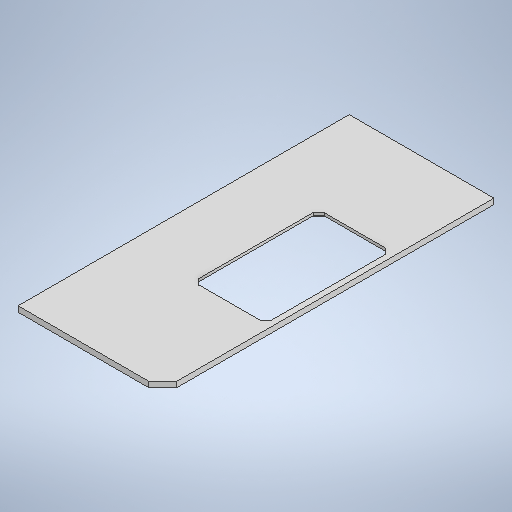
# Autodesk Inventor part: Part6
Saved by Autodesk Inventor 2025.2 (Build 292293000, 293)
## iProperties
Created: 2025-06-06
Part Number: Part6
Material: Generic
Document SubType Name: Sheet Metal
Designer: ziyuz
Density: 1 g/cm^3
Sheet Metal Rule: Default_mm
Appearance: Default
Author: ziyuz
Autodesk Inventor part; units mm, degrees
(part 1 of 2)
ref_plane "YZ Plane" through (0, 0, 0) normal (1, 0, 0) x (0, 1, 0)
ref_plane "XZ Plane" through (0, 0, 0) normal (0, 1, 0) x (-1, 0, 0)
ref_plane "XY Plane" through (0, 0, 0) normal (0, 0, 1) x (1, 0, 0)
sketch "Sketch1" plane through (0, 0, 0) normal (0, 1, 0) x (-1, 0, 0)
  line L0 (-29.0932, -58.6501) -> (-29.0932, -48.6501)
  line L1 (-29.0932, -58.6501) -> (-29.0932, 55.3499)
  line L2 (-29.0932, 55.3499) -> (-24.0932, 60.3499)
  line L3 (-29.0932, 55.3499) -> (-24.0932, 60.3499)
  line L4 (-24.0932, 60.3499) -> (22.9068, 60.3499)
  line L5 (-24.0932, 60.3499) -> (22.9068, 60.3499)
  line L6 (22.9068, 60.3499) -> (22.9068, -58.6501)
  line L7 (22.9068, -58.6501) -> (-29.0932, -58.6501)
  line L8 (-29.0932, -38.6501) -> (0.9068, -38.6501)
  line L9 (-29.0932, -38.6501) -> (2.9068, -38.6501)
  line L10 (2.9068, -38.6501) -> (2.9068, 31.3499)
  line L11 (2.9068, 31.3499) -> (-29.0932, 31.3499)
  line L12 (-29.0932, -38.6501) -> (-29.0932, -23.6501)
  line L13 (-29.0932, -23.6501) -> (2.9068, -23.6501)
  line L14 (-29.0932, 31.3499) -> (-29.0932, 21.3499)
  line L15 (-29.0932, 21.3499) -> (2.9068, 21.3499)
  line L16 (-29.0932, -23.6501) -> (-29.0932, 21.3499)
  line L17 (-29.0932, -23.6501) -> (-27.0932, -23.6501)
  line L18 (-27.0932, -23.6501) -> (-27.0932, 21.3499)
  line L19 (-29.0932, 21.3499) -> (-27.0932, 21.3499)
  line L20 (0.9068, -38.6501) -> (0.9068, 31.3499)
  line L21 (0.9068, -23.6501) -> (-1.0932, -23.6501)
  line L22 (-1.0932, -23.6501) -> (-1.0932, 21.3499)
  point P0 (0, 0)
  point P1 (-27.0932, 58.3499)
  dimension "d0" = 32
  dimension "d1" = 70
  dimension "d2" = 15
  dimension "d3" = 10
  dimension "d4" = 2
  dimension "d5" = 2
  constraints: 46 end point, 11 point on line, 8 perpendicular, 5 collinear, 1 vertical
  measures "d0" distance of L8.start L9.end
  measures "d1" distance of L9.end L10.end
  measures "d2" distance of L8.start L12.end
  measures "d3" distance of L11.end L14.end
  measures "d4" distance of L12.end L17.end
  measures "d5" distance of L21.start L21.end
extrude "Extrusion1" add sketch "Sketch1" along normal blind 2 contours L0 L1 L8 L9 L10 L11 L2 L4 L6 L7 | L1 L13 L20 L8 | L1 L15 L18 L13 | L20 L13 L10 L9 | L1 L11 L20 L15 | L20 L15 L10 L13 | L13 L22 L15 L20 | L20 L11 L10 L15
chamfer "Chamfer1" distance 2 angle 45 4 edges at (27.0932, 1, 21.3499) (27.0932, 1, -23.6501) (1.0932, 1, -23.6501) (1.0932, 1, 21.3499)
chamfer "Chamfer2" distance 1 angle 45 8 edges at (14.0932, 0, -23.6501) (2.0932, 0, -22.6501) (1.0932, 0, -1.1501) (2.0932, 0, 20.3499) (14.0932, 0, 21.3499) (26.0932, 0, 20.3499) (27.0932, 0, -1.1501) (26.0932, 0, -22.6501)
sketch "Sketch2" plane through (0, 0, 0) normal (0, -1, 0) x (1, 0, 0)
  line L0 (22.5848, 53.3001) -> (22.5848, 27.0796) construction
  line L1 (22.5848, 27.0796) -> (14.0309, 27.0796) construction
  line L2 (14.0309, 27.0796) -> (14.0309, 53.3001) construction
  line L3 (14.0309, 53.3001) -> (22.5848, 53.3001) construction
  line L4 (23.1405, -28.7557) -> (23.1405, -54.9763) construction
  line L5 (23.1405, -54.9763) -> (14.5866, -54.9763) construction
  line L6 (14.5866, -54.9763) -> (14.5866, -28.7557) construction
  line L7 (14.5866, -28.7557) -> (23.1405, -28.7557) construction
  line L8 (-13.0132, 54.473) -> (-4.4593, 54.473) construction
  line L9 (-4.4593, 54.473) -> (-4.4593, -53.9023) construction
  line L10 (-4.4593, -53.9023) -> (-13.0132, -53.9023) construction
  line L11 (-13.0132, -53.9023) -> (-13.0132, 54.473) construction
  line L12 (-24.1819, 54.7415) -> (-15.628, 54.7415) construction
  line L13 (-15.628, 54.7415) -> (-15.628, -53.6339) construction
  line L14 (-15.628, -53.6339) -> (-24.1819, -53.6339) construction
  line L15 (-24.1819, -53.6339) -> (-24.1819, 54.7415) construction
  line L16 (16.4848, 43.7144) -> (16.4848, 45.6962)
  line L17 (16.4848, 45.6962) -> (16.8688, 45.6962)
  line L18 (16.8688, 45.6962) -> (16.8688, 45.299)
  spline S0 degree 2 poles (16.8688, 45.299) (16.8688, 45.1621) (16.9571, 45.0739) (17.0586, 45.0739) knots 0 0 0 1 2 2 2
  line L19 (17.0586, 45.0739) -> (21.9095, 45.0739)
  spline S1 degree 2 poles (21.9095, 45.0739) (22.1478, 45.0739) (22.1655, 45.0915) (22.1655, 45.299) knots 0 0 0 1 2 2 2
  spline S2 degree 2 poles (22.1655, 45.299) (22.1655, 45.7448) (21.8565, 46.0846) (21.0576, 46.3804) knots 0 0 0 1 2 2 2
  line L20 (21.0576, 46.3804) -> (21.1105, 46.7379)
  line L21 (21.1105, 46.7379) -> (22.5848, 46.4069)
  line L22 (22.5848, 46.4069) -> (22.5848, 42.9684)
  line L23 (22.5848, 42.9684) -> (21.115, 42.6727)
  line L24 (21.115, 42.6727) -> (21.0576, 42.9949)
  spline S3 degree 2 poles (21.0576, 42.9949) (21.8256, 43.2951) (22.1655, 43.5687) (22.1655, 44.0145) knots 0 0 0 1 2 2 2
  spline S4 degree 2 poles (22.1655, 44.0145) (22.1655, 44.3191) (22.1478, 44.3367) (21.8742, 44.3367) knots 0 0 0 1 2 2 2
  line L25 (21.8742, 44.3367) -> (17.0586, 44.3367)
  spline S5 degree 2 poles (17.0586, 44.3367) (16.9571, 44.3367) (16.8688, 44.2264) (16.8688, 44.1161) knots 0 0 0 1 2 2 2
  line L26 (16.8688, 44.1161) -> (16.8688, 43.7144)
  line L27 (16.8688, 43.7144) -> (16.4848, 43.7144)
  spline S6 degree 2 poles (22.011, 41.7237) (22.1125, 41.7237) (22.2008, 41.812) (22.2008, 41.9488) knots 0 0 0 1 2 2 2
  line L28 (22.2008, 41.9488) -> (22.2008, 42.2446)
  line L29 (22.2008, 42.2446) -> (22.5848, 42.2446)
  line L30 (22.5848, 42.2446) -> (22.5848, 40.5982)
  spline S7 degree 2 poles (22.5848, 40.5982) (22.5848, 39.4859) (21.1414, 38.1529) (19.654, 38.1529) knots 0 0 0 1 2 2 2
  spline S8 degree 2 poles (19.654, 38.1529) (18.0297, 38.1529) (16.4848, 39.4462) (16.4848, 40.7041) knots 0 0 0 1 2 2 2
  line L31 (16.4848, 40.7041) -> (16.4848, 42.2799)
  line L32 (16.4848, 42.2799) -> (16.8688, 42.2799)
  line L33 (16.8688, 42.2799) -> (16.8688, 41.9488)
  spline S9 degree 2 poles (16.8688, 41.9488) (16.8688, 41.812) (16.9571, 41.7237) (17.0586, 41.7237) knots 0 0 0 1 2 2 2
  line L34 (17.0586, 41.7237) -> (22.011, 41.7237)
  spline S10 degree 2 poles (19.5878, 38.9915) (21.0443, 38.9915) (22.2008, 39.8478) (22.2008, 40.5938) knots 0 0 0 1 2 2 2
  spline S11 degree 2 poles (22.2008, 40.5938) (22.2008, 40.81) (22.0993, 40.9866) (22.011, 40.9866) knots 0 0 0 1 2 2 2
  line L35 (22.011, 40.9866) -> (17.0586, 40.9866)
  spline S12 degree 2 poles (17.0586, 40.9866) (16.9659, 40.9866) (16.8688, 40.8454) (16.8688, 40.6997) knots 0 0 0 1 2 2 2
  spline S13 degree 2 poles (16.8688, 40.6997) (16.8688, 39.9802) (17.959, 38.9915) (19.5878, 38.9915) knots 0 0 0 1 2 2 2
  spline S14 degree 2 poles (22.011, 35.403) (22.1125, 35.403) (22.2008, 35.4913) (22.2008, 35.6281) knots 0 0 0 1 2 2 2
  line L36 (22.2008, 35.6281) -> (22.2008, 36.5462)
  line L37 (22.2008, 36.5462) -> (22.5848, 36.5462)
  line L38 (22.5848, 36.5462) -> (22.5848, 33.5227)
  line L39 (22.5848, 33.5227) -> (22.2008, 33.5227)
  line L40 (22.2008, 33.5227) -> (22.2008, 34.4452)
  spline S15 degree 2 poles (22.2008, 34.4452) (22.2008, 34.5511) (22.1125, 34.6659) (22.011, 34.6659) knots 0 0 0 1 2 2 2
  line L41 (22.011, 34.6659) -> (17.0939, 34.6659)
  spline S16 degree 2 poles (17.0939, 34.6659) (16.295, 34.6659) (15.3769, 35.6899) (15.3769, 36.4535) knots 0 0 0 1 2 2 2
  spline S17 degree 2 poles (15.3769, 36.4535) (15.3769, 37.0053) (15.8359, 37.6144) (16.1582, 37.6144) knots 0 0 0 1 2 2 2
  spline S18 degree 2 poles (16.1582, 37.6144) (16.4053, 37.6144) (16.6613, 37.3142) (16.6613, 37.1421) knots 0 0 0 1 2 2 2
  spline S19 degree 2 poles (16.6613, 37.1421) (16.6613, 36.9302) (16.3612, 36.6698) (16.1582, 36.6698) knots 0 0 0 1 2 2 2
  spline S20 degree 2 poles (16.1582, 36.6698) (16.0787, 36.6698) (15.9375, 36.7184) (15.9022, 36.7757) knots 0 0 0 1 2 2 2
  spline S21 degree 2 poles (15.9022, 36.7757) (15.8801, 36.736) (15.7962, 36.5065) (15.7962, 36.3123) knots 0 0 0 1 2 2 2
  spline S22 degree 2 poles (15.7962, 36.3123) (15.7962, 35.9018) (16.3303, 35.403) (17.0939, 35.403) knots 0 0 0 1 2 2 2
  line L42 (17.0939, 35.403) -> (22.011, 35.403)
  line L43 (6.459, 44.9194) -> (6.075, 44.9194)
  line L44 (6.075, 44.9194) -> (6.075, 46.7644)
  line L45 (6.075, 46.7644) -> (6.459, 46.7644)
  line L46 (6.459, 46.7644) -> (6.459, 46.4378)
  spline S23 degree 2 poles (6.459, 46.4378) (6.459, 46.3009) (6.5473, 46.2126) (6.6488, 46.2126) knots 0 0 0 1 2 2 2
  line L47 (6.6488, 46.2126) -> (11.6012, 46.2126)
  spline S24 degree 2 poles (11.6012, 46.2126) (11.7027, 46.2126) (11.791, 46.3009) (11.791, 46.4378) knots 0 0 0 1 2 2 2
  line L48 (11.791, 46.4378) -> (11.791, 46.7335)
  line L49 (11.791, 46.7335) -> (12.175, 46.7335)
  line L50 (12.175, 46.7335) -> (12.175, 42.9773)
  line L51 (12.175, 42.9773) -> (10.789, 42.5359)
  line L52 (10.789, 42.5359) -> (10.6831, 42.8448)
  spline S25 degree 2 poles (10.6831, 42.8448) (11.2657, 43.1494) (11.791, 43.8689) (11.791, 44.2882) knots 0 0 0 1 2 2 2
  line L53 (11.791, 44.2882) -> (11.791, 45.2548)
  spline S26 degree 2 poles (11.791, 45.2548) (11.791, 45.3608) (11.6983, 45.4755) (11.6012, 45.4755) knots 0 0 0 1 2 2 2
  line L54 (11.6012, 45.4755) -> (9.4737, 45.4755)
  line L55 (9.4737, 45.4755) -> (9.4737, 44.4294)
  spline S27 degree 2 poles (9.4737, 44.4294) (9.4737, 44.1205) (9.7341, 43.86) (10.0431, 43.86) knots 0 0 0 1 2 2 2
  line L56 (10.0431, 43.86) -> (10.3035, 43.86)
  line L57 (10.3035, 43.86) -> (10.3035, 43.4716)
  line L58 (10.3035, 43.4716) -> (8.1186, 43.4716)
  line L59 (8.1186, 43.4716) -> (8.1186, 43.86)
  line L60 (8.1186, 43.86) -> (8.3437, 43.86)
  spline S28 degree 2 poles (8.3437, 43.86) (8.7322, 43.86) (9.0897, 44.1293) (9.0897, 44.4294) knots 0 0 0 1 2 2 2
  line L61 (9.0897, 44.4294) -> (9.0897, 45.4755)
  line L62 (9.0897, 45.4755) -> (6.6488, 45.4755)
  spline S29 degree 2 poles (6.6488, 45.4755) (6.5473, 45.4755) (6.459, 45.3608) (6.459, 45.2548) knots 0 0 0 1 2 2 2
  line L63 (6.459, 45.2548) -> (6.459, 44.9194)
  line L64 (8.8469, 40.9513) -> (6.6488, 40.9513)
  spline S30 degree 2 poles (6.6488, 40.9513) (6.5473, 40.9513) (6.459, 40.8365) (6.459, 40.7306) knots 0 0 0 1 2 2 2
  line L65 (6.459, 40.7306) -> (6.459, 40.3951)
  line L66 (6.459, 40.3951) -> (6.075, 40.3951)
  line L67 (6.075, 40.3951) -> (6.075, 42.2401)
  line L68 (6.075, 42.2401) -> (6.459, 42.2401)
  line L69 (6.459, 42.2401) -> (6.459, 41.9135)
  spline S31 degree 2 poles (6.459, 41.9135) (6.459, 41.7767) (6.5473, 41.6884) (6.6488, 41.6884) knots 0 0 0 1 2 2 2
  line L70 (6.6488, 41.6884) -> (11.6012, 41.6884)
  spline S32 degree 2 poles (11.6012, 41.6884) (11.7027, 41.6884) (11.791, 41.7767) (11.791, 41.9135) knots 0 0 0 1 2 2 2
  line L71 (11.791, 41.9135) -> (11.791, 42.2092)
  line L72 (11.791, 42.2092) -> (12.175, 42.2092)
  line L73 (12.175, 42.2092) -> (12.175, 40.0773)
  spline S33 degree 2 poles (12.175, 40.0773) (12.175, 39.1769) (11.2569, 38.1838) (10.5639, 38.1838) knots 0 0 0 1 2 2 2
  spline S34 degree 2 poles (10.5639, 38.1838) (9.7253, 38.1838) (8.8469, 39.2431) (8.8469, 39.9714) knots 0 0 0 1 2 2 2
  line L74 (8.8469, 39.9714) -> (8.8469, 40.9513)
  spline S35 degree 2 poles (9.2309, 40.1789) (9.2309, 39.6889) (9.8092, 38.9518) (10.5286, 38.9518) knots 0 0 0 1 2 2 2
  spline S36 degree 2 poles (10.5286, 38.9518) (11.1819, 38.9518) (11.791, 39.5609) (11.791, 40.2495) knots 0 0 0 1 2 2 2
  line L75 (11.791, 40.2495) -> (11.791, 40.7306)
  spline S37 degree 2 poles (11.791, 40.7306) (11.791, 40.8365) (11.6983, 40.9513) (11.6012, 40.9513) knots 0 0 0 1 2 2 2
  line L76 (11.6012, 40.9513) -> (9.2309, 40.9513)
  line L77 (9.2309, 40.9513) -> (9.2309, 40.1789)
  line L78 (6.075, 34.6659) -> (6.075, 36.6477)
  line L79 (6.075, 36.6477) -> (6.459, 36.6477)
  line L80 (6.459, 36.6477) -> (6.459, 36.2505)
  spline S38 degree 2 poles (6.459, 36.2505) (6.459, 36.1137) (6.5473, 36.0254) (6.6488, 36.0254) knots 0 0 0 1 2 2 2
  line L81 (6.6488, 36.0254) -> (11.4997, 36.0254)
  spline S39 degree 2 poles (11.4997, 36.0254) (11.738, 36.0254) (11.7557, 36.043) (11.7557, 36.2505) knots 0 0 0 1 2 2 2
  spline S40 degree 2 poles (11.7557, 36.2505) (11.7557, 36.6963) (11.4467, 37.0362) (10.6478, 37.3319) knots 0 0 0 1 2 2 2
  line L82 (10.6478, 37.3319) -> (10.7008, 37.6894)
  line L83 (10.7008, 37.6894) -> (12.175, 37.3584)
  line L84 (12.175, 37.3584) -> (12.175, 33.92)
  line L85 (12.175, 33.92) -> (10.7052, 33.6242)
  line L86 (10.7052, 33.6242) -> (10.6478, 33.9464)
  spline S41 degree 2 poles (10.6478, 33.9464) (11.4158, 34.2466) (11.7557, 34.5202) (11.7557, 34.9661) knots 0 0 0 1 2 2 2
  spline S42 degree 2 poles (11.7557, 34.9661) (11.7557, 35.2706) (11.738, 35.2883) (11.4644, 35.2883) knots 0 0 0 1 2 2 2
  line L87 (11.4644, 35.2883) -> (6.6488, 35.2883)
  spline S43 degree 2 poles (6.6488, 35.2883) (6.5473, 35.2883) (6.459, 35.1779) (6.459, 35.0676) knots 0 0 0 1 2 2 2
  line L88 (6.459, 35.0676) -> (6.459, 34.6659)
  line L89 (6.459, 34.6659) -> (6.075, 34.6659)
  point P0 (0, 0)
  constraints: 8 other
extrude "Extrusion2" add sketch "Sketch2" along normal blind 0.5
sketch "Sketch4" plane through (0, 0, 0) normal (0, -1, 0) x (1, 0, 0)
  line L0 (23.6842, -29.6175) -> (23.6842, -52.515) construction
  line L1 (23.6842, -52.515) -> (1.0923, -52.515) construction
  line L2 (1.0923, -52.515) -> (1.0923, -29.6175) construction
  line L3 (1.0923, -29.6175) -> (23.6842, -29.6175) construction
  spline S0 degree 2 poles (18.1434, -33.7347) (18.3329, -33.7347) (18.5408, -33.9796) (18.5408, -34.3262) (18.4761, -34.6543) (18.3699, -34.7976) knots 0 0 0 1 2 3 4 4 4
  line L4 (18.3699, -34.7976) -> (18.3699, -35.1765)
  spline S1 degree 2 poles (18.3699, -35.1765) (18.3606, -35.2967) (18.3606, -35.403) knots 0 0 0 1 1 1
  line L5 (18.3606, -35.403) -> (18.3606, -35.5555)
  spline S2 degree 2 poles (18.3606, -35.5555) (18.3606, -35.7496) (18.3375, -36.2764) (18.393, -36.8078) (18.5639, -37.2792) (18.7627, -37.4224) knots 0 0 0 1 2 3 4 4 4
  spline S3 degree 2 poles (18.7627, -37.4224) (18.7072, -37.3716) (18.7026, -37.2653) (18.7026, -37.196) knots 0 0 0 1 2 2 2
  line L6 (18.7026, -37.196) -> (18.7026, -37.0851)
  line L7 (18.7026, -37.0851) -> (18.7534, -36.9187)
  spline S4 degree 2 poles (18.7534, -36.9187) (18.7904, -36.7986) (18.8828, -36.5352) (18.929, -36.415) knots 0 0 0 1 2 2 2
  line L8 (18.929, -36.415) -> (18.9799, -36.2487)
  spline S5 degree 2 poles (18.9799, -36.2487) (18.9937, -36.2117) (19.1, -35.976) (19.1693, -35.842) knots 0 0 0 1 2 2 2
  line L9 (19.1693, -35.842) -> (19.2895, -35.5832)
  spline S6 degree 2 poles (19.2895, -35.5832) (19.3403, -35.463) (19.3727, -35.4122) knots 0 0 0 1 1 1
  spline S7 degree 2 poles (19.3727, -35.4122) (19.3865, -35.3799) (19.4928, -35.1996) (19.6222, -34.9824) (19.7331, -34.793) (19.7655, -34.7468) knots 0 0 0 1 2 3 4 4 4
  spline S8 degree 2 poles (19.7655, -34.7468) (19.8302, -34.6312) (20.052, -34.3262) (20.3154, -34.0443) (20.6065, -33.8502) (20.7683, -33.8502) knots 0 0 0 1 2 3 4 4 4
  spline S9 degree 2 poles (20.7683, -33.8502) (20.9947, -33.8502) (21.2442, -34.1414) (21.272, -34.354) knots 0 0 0 1 2 2 2
  spline S10 degree 2 poles (21.272, -34.354) (21.2812, -34.4094) (21.2951, -34.5573) knots 0 0 0 1 1 1
  line L10 (21.2951, -34.5573) -> (21.3321, -34.9224)
  spline S11 degree 2 poles (21.3321, -34.9224) (21.3459, -35.1303) (21.3783, -35.3706) knots 0 0 0 1 1 1
  line L11 (21.3783, -35.3706) -> (21.4245, -35.842)
  spline S12 degree 2 poles (21.4245, -35.842) (21.4383, -36.073) (21.4753, -36.4659) (21.5077, -36.7062) (21.711, -36.8818) (21.8311, -36.9187) knots 0 0 0 1 2 3 4 4 4
  line L12 (21.8311, -36.9187) -> (22.8339, -37.7043)
  spline S13 degree 2 poles (22.8339, -37.7043) (22.8709, -37.7413) (22.9033, -37.8984) (22.9033, -37.9446) knots 0 0 0 1 2 2 2
  spline S14 degree 2 poles (22.9033, -37.9446) (22.6907, -37.9446) (22.3349, -37.7644) (22.0206, -37.5426) (21.7572, -37.3624) (21.6324, -37.3624) knots 0 0 0 1 2 3 4 4 4
  spline S15 degree 2 poles (21.6324, -37.3624) (21.5816, -37.3624) (21.5492, -37.4224) knots 0 0 0 1 1 1
  spline S16 degree 2 poles (21.5492, -37.4224) (21.5677, -37.2884) (21.3783, -37.1359) (21.138, -37.0158) (20.9254, -36.8679) (20.9254, -36.7293) knots 0 0 0 1 2 3 4 4 4
  spline S17 degree 2 poles (20.9254, -36.7293) (20.9254, -36.6415) (20.9947, -36.5814) (21.1056, -36.5814) (21.2489, -36.6091) (21.3228, -36.6091) knots 0 0 0 1 2 3 4 4 4
  line L13 (21.3228, -36.6091) -> (21.3228, -36.5259)
  line L14 (21.3228, -36.5259) -> (20.8191, -34.7468)
  spline S18 degree 2 poles (20.8191, -34.7468) (20.7498, -34.6867) (20.6389, -34.5434) (20.6019, -34.4695) knots 0 0 0 1 2 2 2
  spline S19 degree 2 poles (20.6019, -34.4695) (20.5095, -34.5896) (20.3154, -34.8762) (20.1352, -35.1858) (19.9734, -35.4862) (19.9318, -35.6387) knots 0 0 0 1 2 3 4 4 4
  spline S20 degree 2 poles (19.9318, -35.6387) (19.8717, -35.8189) (19.7424, -36.2255) (19.5806, -36.623) (19.3865, -36.9927) (19.2571, -37.1452) knots 0 0 0 1 2 3 4 4 4
  spline S21 degree 2 poles (19.2571, -37.1452) (19.2063, -37.2052) (19.0538, -37.4086) (18.8874, -37.6119) (18.7072, -37.7644) (18.624, -37.7644) knots 0 0 0 1 2 3 4 4 4
  spline S22 degree 2 poles (18.624, -37.7644) (18.4068, -37.7644) (18.1942, -37.538) (18.0649, -37.2376) (17.9447, -36.9418) (17.8107, -36.8679) knots 0 0 0 1 2 3 4 4 4
  spline S23 degree 2 poles (17.8107, -36.8679) (17.6074, -36.3734) (17.4179, -35.3568) (17.4179, -34.8299) knots 0 0 0 1 2 2 2
  spline S24 degree 2 poles (17.4179, -34.8299) (17.4179, -34.6266) (17.4641, -34.2338) (17.6212, -33.9242) (17.9031, -33.7347) (18.1434, -33.7347) knots 0 0 0 1 2 3 4 4 4
  spline S25 degree 2 poles (21.8358, -38.9705) (21.882, -38.9798) (22.0483, -39.0168) knots 0 0 0 1 1 1
  line L15 (22.0483, -39.0168) -> (22.4088, -39.1138)
  spline S26 degree 2 poles (22.4088, -39.1138) (22.6075, -39.1739) (22.9772, -39.2802) (23.065, -39.3079) knots 0 0 0 1 2 2 2
  line L16 (23.065, -39.3079) -> (23.1482, -39.3495)
  spline S27 degree 2 poles (23.1482, -39.3495) (23.2267, -39.3865) (23.3099, -39.4234) knots 0 0 0 1 1 1
  line L17 (23.3099, -39.4234) -> (23.4902, -39.5159)
  spline S28 degree 2 poles (23.4902, -39.5159) (23.578, -39.5574) (23.6704, -39.6129) (23.6842, -39.6591) (23.6842, -39.7007) knots 0 0 0 1 2 3 3 3
  spline S29 degree 2 poles (23.6842, -39.7007) (23.6842, -39.7099) (23.6796, -39.7238) knots 0 0 0 1 1 1
  line L18 (23.6796, -39.7238) -> (23.6796, -39.7562)
  spline S30 degree 2 poles (23.6796, -39.7562) (23.5641, -39.8209) (23.2406, -39.8902) (22.9171, -39.9225) (22.76, -39.9225) knots 0 0 0 1 2 3 3 3
  line L19 (22.76, -39.9225) -> (22.5105, -39.9225)
  spline S31 degree 2 poles (22.5105, -39.9225) (22.4319, -39.9502) (22.2886, -40.0473) (22.2286, -40.0889) knots 0 0 0 1 2 2 2
  line L20 (22.2286, -40.0889) -> (18.9429, -41.7063)
  spline S32 degree 2 poles (18.9429, -41.7063) (18.9336, -41.808) (18.9336, -41.979) (18.8967, -42.0945) (18.8042, -42.1592) (18.7164, -42.1592) knots 0 0 0 1 2 3 4 4 4
  spline S33 degree 2 poles (18.7164, -42.1592) (18.6471, -42.1592) (18.5778, -42.0991) (18.5593, -42.0621) knots 0 0 0 1 2 2 2
  line L21 (18.5593, -42.0621) -> (18.5131, -42.0021)
  spline S34 degree 2 poles (18.5131, -42.0021) (18.49, -41.979) (18.4346, -41.979) knots 0 0 0 1 1 1
  spline S35 degree 2 poles (18.4346, -41.979) (18.2867, -41.979) (18.0048, -42.0945) (17.7136, -42.2377) (17.4086, -42.3487) (17.2469, -42.3487) knots 0 0 0 1 2 3 4 4 4
  spline S36 degree 2 poles (17.2469, -42.3487) (17.2469, -42.2886) (17.2515, -42.1361) (17.3208, -42.0991) knots 0 0 0 1 2 2 2
  line L22 (17.3208, -42.0991) -> (18.5501, -41.4799)
  spline S37 degree 2 poles (18.5501, -41.4799) (18.5593, -41.1333) (18.5732, -40.8098) knots 0 0 0 1 1 1
  line L23 (18.5732, -40.8098) -> (18.5871, -40.2368)
  spline S38 degree 2 poles (18.5871, -40.2368) (18.5963, -39.9502) (18.6009, -39.7562) knots 0 0 0 1 1 1
  line L24 (18.6009, -39.7562) -> (18.6009, -39.5297)
  spline S39 degree 2 poles (18.6009, -39.5297) (18.5131, -39.4974) (18.1942, -39.4696) (17.8246, -39.4234) (17.4317, -39.3541) (17.1221, -39.2432) (16.9188, -39.063) (16.9188, -38.9243) knots 0 0 0 1 2 3 4 5 6 6 6
  spline S40 degree 2 poles (16.9188, -38.9243) (16.9188, -38.8735) (16.965, -38.7349) (17.0436, -38.6101) (17.1452, -38.5269) (17.2053, -38.5269) knots 0 0 0 1 2 3 4 4 4
  line L25 (17.2053, -38.5269) -> (18.49, -38.5269)
  line L26 (18.49, -38.5269) -> (21.8358, -38.9705)
  line L27 (18.9198, -39.5898) -> (18.9198, -39.9826)
  spline S41 degree 2 poles (18.9198, -39.9826) (18.9198, -40.1905) (18.9336, -40.6388) (18.966, -41.0732) (18.9937, -41.2627) knots 0 0 0 1 2 3 3 3
  line L28 (18.9937, -41.2627) -> (19.3264, -41.1518)
  line L29 (19.3264, -41.1518) -> (22.0576, -39.8763)
  line L30 (22.0576, -39.8763) -> (19.2155, -39.5898)
  line L31 (19.2155, -39.5898) -> (18.9198, -39.5898)
  spline S42 degree 2 poles (17.2977, -44.0909) (17.3717, -44.0585) (17.538, -44.0077) knots 0 0 0 1 1 1
  line L32 (17.538, -44.0077) -> (17.917, -43.8829)
  line L33 (17.917, -43.8829) -> (18.3514, -43.7581)
  spline S43 degree 2 poles (18.3514, -43.7581) (18.5778, -43.6888) (19.003, -43.5779) (19.3357, -43.4855) (19.4189, -43.4716) knots 0 0 0 1 2 3 3 3
  line L34 (19.4189, -43.4716) -> (19.8255, -43.3884)
  line L35 (19.8255, -43.3884) -> (20.3662, -43.2914)
  spline S44 degree 2 poles (20.3662, -43.2914) (20.662, -43.2452) (21.2627, -43.1481) (21.7849, -43.0696) (22.1546, -43.0234) (22.2055, -43.0234) knots 0 0 0 1 2 3 4 4 4
  line L36 (22.2055, -43.0234) -> (22.5983, -43.0234)
  spline S45 degree 2 poles (22.5983, -43.0234) (22.6445, -43.0234) (22.7138, -43.1666) (22.7508, -43.3561) (22.7646, -43.5455) (22.7646, -43.5825) knots 0 0 0 1 2 3 4 4 4
  line L37 (22.7646, -43.5825) -> (22.7646, -43.638)
  spline S46 degree 2 poles (22.7646, -43.638) (22.6445, -43.6796) (22.2655, -43.7627) (21.8912, -43.8459) (21.5585, -43.9522) (21.4846, -44.0308) knots 0 0 0 1 2 3 4 4 4
  line L38 (21.4846, -44.0308) -> (19.1, -46.4708)
  line L39 (19.1, -46.4708) -> (20.9254, -47.0438)
  spline S47 degree 2 poles (20.9254, -47.0438) (21.0086, -47.1039) (21.4152, -47.2333) (21.9189, -47.3858) (22.4735, -47.5337) (22.9217, -47.6862) (23.2175, -47.8387) (23.2175, -47.9034) knots 0 0 0 1 2 3 4 5 6 6 6
  spline S48 degree 2 poles (23.2175, -47.9034) (23.2175, -47.9449) (23.2083, -48.0327) (23.1574, -48.0466) knots 0 0 0 1 2 2 2
  line L40 (23.1574, -48.0466) -> (22.3718, -48.1621)
  spline S49 degree 2 poles (22.3718, -48.1621) (21.7387, -48.1529) (21.1426, -48.1621) knots 0 0 0 1 1 1
  line L41 (21.1426, -48.1621) -> (19.9503, -48.176)
  spline S50 degree 2 poles (19.9503, -48.176) (19.3634, -48.1899) (18.1942, -48.213) (17.5842, -48.213) knots 0 0 0 1 2 2 2
  spline S51 degree 2 poles (17.5842, -48.213) (17.5011, -48.213) (17.3486, -48.1852) (17.2977, -48.1021) knots 0 0 0 1 2 2 2
  spline S52 degree 2 poles (17.2977, -48.1021) (17.2885, -48.079) (17.2839, -47.9265) (17.2839, -47.9034) knots 0 0 0 1 2 2 2
  spline S53 degree 2 poles (17.2839, -47.9034) (17.2839, -47.8664) (17.2885, -47.7185) (17.2977, -47.7093) knots 0 0 0 1 2 2 2
  spline S54 degree 2 poles (17.2977, -47.7093) (17.307, -47.6862) (17.3671, -47.6122) (17.404, -47.5752) knots 0 0 0 1 2 2 2
  line L42 (17.404, -47.5752) -> (17.478, -47.5105)
  spline S55 degree 2 poles (17.478, -47.5105) (17.5103, -47.4921) (17.5242, -47.4921) knots 0 0 0 1 1 1
  line L43 (17.5242, -47.4921) -> (20.5326, -47.4921)
  line L44 (20.5326, -47.4921) -> (20.4817, -47.432)
  line L45 (20.4817, -47.432) -> (18.5778, -46.8728)
  spline S56 degree 2 poles (18.5778, -46.8728) (18.4946, -46.8497) (18.3514, -46.7296) (18.3514, -46.6325) knots 0 0 0 1 2 2 2
  spline S57 degree 2 poles (18.3514, -46.6325) (18.3514, -46.5863) (18.3699, -46.4662) (18.4161, -46.4246) knots 0 0 0 1 2 2 2
  spline S58 degree 2 poles (18.4161, -46.4246) (18.4207, -46.4199) (18.4761, -46.3876) knots 0 0 0 1 1 1
  line L46 (18.4761, -46.3876) -> (18.5778, -46.3368)
  line L47 (18.5778, -46.3368) -> (18.6841, -46.2905)
  line L48 (18.6841, -46.2905) -> (18.7442, -46.2628)
  spline S59 degree 2 poles (18.7442, -46.2628) (18.7534, -46.2628) (18.7904, -46.2166) (18.8042, -46.2074) knots 0 0 0 1 2 2 2
  spline S60 degree 2 poles (18.8042, -46.2074) (19.0399, -45.9209) (19.5621, -45.4079) (19.8302, -45.1584) knots 0 0 0 1 2 2 2
  line L49 (19.8302, -45.1584) -> (20.3616, -44.6639)
  spline S61 degree 2 poles (20.3616, -44.6639) (20.625, -44.4143) (20.8653, -44.1417) knots 0 0 0 1 1 1
  line L50 (20.8653, -44.1417) -> (20.759, -44.1417)
  line L51 (20.759, -44.1417) -> (19.9827, -44.2988)
  spline S62 degree 2 poles (19.9827, -44.2988) (19.576, -44.3912) (18.7211, -44.5391) (17.8708, -44.6454) (17.4641, -44.6454) knots 0 0 0 1 2 3 3 3
  line L52 (17.4641, -44.6454) -> (17.2469, -44.6454)
  spline S63 degree 2 poles (17.2469, -44.6454) (17.1406, -44.6177) (17.1175, -44.4652) (17.1175, -44.3912) knots 0 0 0 1 2 2 2
  spline S64 degree 2 poles (17.1175, -44.3912) (17.1175, -44.2849) (17.1683, -44.1324) (17.2977, -44.0909) knots 0 0 0 1 2 2 2
  line L53 (20.6851, -48.5365) -> (20.5696, -48.5365)
  line L54 (20.5696, -48.5365) -> (20.5696, -48.4348)
  line L55 (20.5696, -48.4348) -> (20.6851, -48.4348)
  line L56 (20.6851, -48.4348) -> (20.6851, -48.5365)
  line L57 (22.5983, -46.4246) -> (22.5382, -46.4246)
  line L58 (22.5382, -46.4246) -> (22.5382, -46.2628)
  line L59 (22.5382, -46.2628) -> (22.5983, -46.2628)
  line L60 (22.5983, -46.2628) -> (22.5983, -46.4246)
  spline S65 degree 2 poles (6.4292, -34.3748) (6.42, -34.2777) (6.4385, -33.871) (6.4893, -33.4551) (6.5817, -33.1409) (6.6464, -33.1409) knots 0 0 0 1 2 3 4 4 4
  spline S66 degree 2 poles (6.6464, -33.1409) (6.7666, -33.1409) (6.8729, -33.3904) (6.8729, -33.4875) knots 0 0 0 1 2 2 2
  spline S67 degree 2 poles (6.8729, -33.4875) (7.0993, -33.6123) (7.4551, -33.8618) (7.6215, -33.9912) knots 0 0 0 1 2 2 2
  line L61 (7.6215, -33.9912) -> (7.9542, -34.2638)
  spline S68 degree 2 poles (7.9542, -34.2638) (8.116, -34.3979) (8.3285, -34.5411) knots 0 0 0 1 1 1
  spline S69 degree 2 poles (8.3285, -34.5411) (8.8554, -34.9062) (9.8997, -35.6594) (10.4497, -35.9968) knots 0 0 0 1 2 2 2
  line L62 (10.4497, -35.9968) -> (10.4497, -35.8258)
  line L63 (10.4497, -35.8258) -> (10.0014, -33.3719)
  line L64 (10.0014, -33.3719) -> (10.0014, -33.1455)
  spline S70 degree 2 poles (10.0014, -33.1455) (10.0476, -33.1779) (10.1262, -33.3211) (10.177, -33.4782) (10.2001, -33.5476) knots 0 0 0 1 2 3 3 3
  line L65 (10.2001, -33.5476) -> (10.2232, -33.6538)
  line L66 (10.2232, -33.6538) -> (10.2232, -33.3119)
  line L67 (10.2232, -33.3119) -> (11.0088, -36.3295)
  spline S71 degree 2 poles (11.0088, -36.3295) (11.0597, -36.4035) (11.2353, -36.6669) (11.4063, -36.9719) (11.5264, -37.2815) (11.5264, -37.3924) knots 0 0 0 1 2 3 4 4 4
  line L68 (11.5264, -37.3924) -> (11.2861, -37.3924)
  line L69 (11.2861, -37.3924) -> (6.8497, -34.4117)
  line L70 (6.8497, -34.4117) -> (6.5956, -37.6697)
  line L71 (6.5956, -37.6697) -> (6.5956, -37.7159)
  line L72 (6.5956, -37.7159) -> (6.5817, -37.8083)
  spline S72 degree 2 poles (6.5817, -37.8083) (6.5632, -37.8545) (6.5216, -37.9377) (6.4893, -37.9516) knots 0 0 0 1 2 2 2
  line L73 (6.4893, -37.9516) -> (6.3738, -38.5107)
  line L74 (6.3738, -38.5107) -> (6.0364, -38.5107)
  spline S73 degree 2 poles (6.0364, -38.5107) (6.0364, -37.4848) (6.2536, -35.3637) (6.4292, -34.3748) knots 0 0 0 1 2 2 2
  spline S74 degree 2 poles (11.5588, -33.1455) (11.5588, -33.2888) (11.5033, -33.4274) (11.3554, -33.4274) knots 0 0 0 1 2 2 2
  spline S75 degree 2 poles (11.3554, -33.4274) (11.3554, -33.3211) (11.4294, -33.1455) (11.5588, -33.1455) knots 0 0 0 1 2 2 2
  spline S76 degree 2 poles (6.0595, -43.1181) (6.1335, -43.0118) (6.2536, -43.0072) knots 0 0 0 1 1 1
  line L75 (6.2536, -43.0072) -> (6.48, -43.0072)
  spline S77 degree 2 poles (6.48, -43.0072) (6.956, -43.0072) (7.8988, -43.0673) (8.3747, -43.0673) knots 0 0 0 1 2 2 2
  line L76 (8.3747, -43.0673) -> (8.7352, -43.0673)
  spline S78 degree 2 poles (8.7352, -43.0673) (8.6936, -42.8916) (8.6382, -42.5959) (8.6243, -42.3094) (8.6243, -42.1615) knots 0 0 0 1 2 3 3 3
  line L77 (8.6243, -42.1615) -> (8.6243, -41.8426)
  spline S79 degree 2 poles (8.6243, -41.8426) (8.6243, -41.4591) (8.7352, -40.7104) (8.7352, -40.3269) knots 0 0 0 1 2 2 2
  line L78 (8.7352, -40.3269) -> (8.6844, -40.3269)
  line L79 (8.6844, -40.3269) -> (6.6788, -40.8352)
  line L80 (6.6788, -40.8352) -> (6.1196, -40.8352)
  spline S80 degree 2 poles (6.1196, -40.8352) (6.0688, -40.8352) (5.9671, -40.6966) (5.8839, -40.5256) (5.8331, -40.35) (5.8331, -40.3223) knots 0 0 0 1 2 3 4 4 4
  spline S81 degree 2 poles (5.8331, -40.3223) (5.8331, -40.2298) (5.8793, -40.0866) (6.0087, -40.0496) knots 0 0 0 1 2 2 2
  line L81 (6.0087, -40.0496) -> (9.6872, -39.0976)
  spline S82 degree 2 poles (9.6872, -39.0976) (9.6964, -39.0976) (9.7981, -39.0838) knots 0 0 0 1 1 1
  line L82 (9.7981, -39.0838) -> (10.0338, -39.0468)
  line L83 (10.0338, -39.0468) -> (10.3064, -39.0144)
  spline S83 degree 2 poles (10.3064, -39.0144) (10.4404, -39.0006) (10.5236, -38.9913) knots 0 0 0 1 1 1
  spline S84 degree 2 poles (10.5236, -38.9913) (10.5329, -38.9913) (10.556, -38.9867) knots 0 0 0 1 1 1
  line L84 (10.556, -38.9867) -> (10.7824, -38.9867)
  spline S85 degree 2 poles (10.7824, -38.9867) (10.9164, -38.9867) (11.2122, -39.0329) (11.4294, -39.1346) (11.4294, -39.2409) knots 0 0 0 1 2 3 3 3
  spline S86 degree 2 poles (11.4294, -39.2409) (11.4294, -39.3102) (11.226, -39.4673) (10.9164, -39.6198) (10.5329, -39.7631) (10.1678, -39.8832) (10.0245, -39.9294) knots 0 0 0 1 2 3 4 5 5 5
  line L85 (10.0245, -39.9294) -> (9.7981, -39.9941)
  spline S87 degree 2 poles (9.7981, -39.9941) (9.7565, -40.0126) (9.5347, -40.0727) (9.2851, -40.1374) (9.0587, -40.2021) (9.0171, -40.216) knots 0 0 0 1 2 3 4 4 4
  line L86 (9.0171, -40.216) -> (9.0171, -41.6716)
  spline S88 degree 2 poles (9.0171, -41.6716) (9.0079, -41.875) (9.0171, -42.2354) (9.0448, -42.6051) (9.0772, -42.8408) knots 0 0 0 1 2 3 3 3
  spline S89 degree 2 poles (9.0772, -42.8408) (9.0818, -42.8916) (9.1234, -43.0673) (9.128, -43.0673) knots 0 0 0 1 2 2 2
  line L87 (9.128, -43.0673) -> (11.0273, -43.1782)
  spline S90 degree 2 poles (11.0273, -43.1782) (11.1429, -43.1874) (11.3369, -43.2613) (11.5264, -43.3676) (11.7066, -43.4739) (11.91, -43.5479) (12.0994, -43.5617) (12.2381, -43.6033) (12.3213, -43.6819) (12.3213, -43.7974) knots 0 0 0 1 2 3 4 5 6 7 8 8 8
  spline S91 degree 2 poles (12.3213, -43.7974) (12.3213, -43.8436) (12.2982, -43.9869) (12.1965, -43.9545) knots 0 0 0 1 2 2 2
  line L88 (12.1965, -43.9545) -> (11.7852, -43.9545)
  spline S92 degree 2 poles (11.7852, -43.9545) (11.6466, -43.9638) (11.5264, -43.9638) knots 0 0 0 1 1 1
  line L89 (11.5264, -43.9638) -> (11.1567, -43.9638)
  spline S93 degree 2 poles (11.1567, -43.9638) (11.0227, -43.9638) (10.8841, -43.9545) knots 0 0 0 1 1 1
  line L90 (10.8841, -43.9545) -> (10.5236, -43.9545)
  line L91 (10.5236, -43.9545) -> (9.9737, -43.9314)
  spline S94 degree 2 poles (9.9737, -43.9314) (9.5947, -43.9176) (8.6474, -43.8713) (7.6076, -43.8298) (6.6557, -43.7835) (6.286, -43.7604) knots 0 0 0 1 2 3 4 4 4
  line L92 (6.286, -43.7604) -> (5.7268, -43.7373)
  spline S95 degree 2 poles (5.7268, -43.7373) (5.5789, -43.6911) (5.3894, -43.5941) (5.3894, -43.4277) knots 0 0 0 1 2 2 2
  spline S96 degree 2 poles (5.3894, -43.4277) (5.3894, -43.2983) (5.5235, -43.1782) (5.7222, -43.1273) (5.9532, -43.1273) (6.0595, -43.1181) knots 0 0 0 1 2 3 4 4 4
  line L93 (6.956, -38.9313) -> (6.8451, -38.9313)
  line L94 (6.8451, -38.9313) -> (6.8451, -38.8204)
  line L95 (6.8451, -38.8204) -> (6.956, -38.8204)
  line L96 (6.956, -38.8204) -> (6.956, -38.9313)
  line L97 (10.9072, -44.3381) -> (10.8009, -44.3381)
  line L98 (10.8009, -44.3381) -> (10.8009, -44.2272)
  line L99 (10.8009, -44.2272) -> (10.9072, -44.2272)
  line L100 (10.9072, -44.2272) -> (10.9072, -44.3381)
  spline S97 degree 2 poles (11.1429, -42.1153) (11.129, -42.1384) (11.0874, -42.1384) (11.0735, -42.0922) (11.1521, -42.0922) (11.1429, -42.1153) knots 0 0 0 1 2 3 4 4 4
  spline S98 degree 2 poles (6.1427, -44.0469) (6.1427, -44.0608) (6.0826, -44.0608) (6.0826, -44.0238) (6.1427, -44.0238) (6.1427, -44.0469) knots 0 0 0 1 2 3 4 4 4
  spline S99 degree 2 poles (6.4431, -48.4048) (6.2721, -48.0304) (6.1057, -47.2448) (6.1057, -46.8289) knots 0 0 0 1 2 2 2
  line L101 (6.1057, -46.8289) -> (6.1057, -46.6718)
  spline S100 degree 2 poles (6.1057, -46.6718) (6.0965, -46.5748) (6.1104, -46.3714) (6.1658, -46.1727) (6.2259, -46.1219) knots 0 0 0 1 2 3 3 3
  spline S101 degree 2 poles (6.2259, -46.1219) (6.2536, -46.0895) (6.3969, -45.9601) (6.5586, -45.8169) (6.7019, -45.6967) (6.7527, -45.6505) (6.9191, -45.5719) (6.9514, -45.5627) knots 0 0 0 1 2 3 4 5 6 6 6
  line L102 (6.9514, -45.5627) -> (9.8443, -44.8926)
  spline S102 degree 2 poles (9.8443, -44.8926) (10.0661, -44.8372) (10.3341, -44.8326) knots 0 0 0 1 1 1
  line L103 (10.3341, -44.8326) -> (11.0597, -44.8326)
  spline S103 degree 2 poles (11.0597, -44.8326) (11.1336, -44.8372) (11.2029, -44.8372) knots 0 0 0 1 1 1
  line L104 (11.2029, -44.8372) -> (11.3, -44.8372)
  spline S104 degree 2 poles (11.3, -44.8372) (11.3462, -44.8557) (11.36, -44.9065) (11.36, -44.9435) knots 0 0 0 1 2 2 2
  spline S105 degree 2 poles (11.36, -44.9435) (11.36, -45.0174) (11.3138, -45.2901) (11.166, -45.3871) (10.9395, -45.4657) (10.6992, -45.5073) (10.4728, -45.5488) (10.4035, -45.5627) knots 0 0 0 1 2 3 4 5 6 6 6
  spline S106 degree 2 poles (10.4035, -45.5627) (9.7149, -45.7198) (8.3609, -46.0618) (7.6723, -46.2328) knots 0 0 0 1 2 2 2
  spline S107 degree 2 poles (7.6723, -46.2328) (7.6492, -46.242) (7.5845, -46.2559) knots 0 0 0 1 1 1
  line L105 (7.5845, -46.2559) -> (7.4228, -46.2882)
  spline S108 degree 2 poles (7.4228, -46.2882) (7.335, -46.3067) (7.1917, -46.3391) (7.1363, -46.3529) (7.0716, -46.3853) knots 0 0 0 1 2 3 3 3
  line L106 (7.0716, -46.3853) -> (6.9191, -46.4454)
  line L107 (6.9191, -46.4454) -> (6.7666, -46.5147)
  spline S109 degree 2 poles (6.7666, -46.5147) (6.6926, -46.5516) (6.6695, -46.5655) knots 0 0 0 1 1 1
  spline S110 degree 2 poles (6.6695, -46.5655) (6.6649, -46.5932) (6.6557, -46.7596) (6.6557, -46.7919) knots 0 0 0 1 2 2 2
  spline S111 degree 2 poles (6.6557, -46.7919) (6.6557, -46.9491) (6.725, -47.3927) (6.8682, -47.8456) (7.0762, -48.2476) (7.2287, -48.3539) knots 0 0 0 1 2 3 4 4 4
  line L108 (7.2287, -48.3539) -> (7.5614, -48.3539)
  spline S112 degree 2 poles (7.5614, -48.3539) (8.1021, -48.3539) (9.1742, -48.2938) (9.7149, -48.2938) knots 0 0 0 1 2 2 2
  line L109 (9.7149, -48.2938) -> (10.653, -48.2938)
  spline S113 degree 2 poles (10.653, -48.2938) (10.7824, -48.2985) (10.7963, -48.2985) knots 0 0 0 1 1 1
  line L110 (10.7963, -48.2985) -> (10.9672, -48.2985)
  spline S114 degree 2 poles (10.9672, -48.2985) (11.0874, -48.3077) (11.3369, -48.3585) (11.5264, -48.4787) (11.5264, -48.6035) knots 0 0 0 1 2 3 3 3
  spline S115 degree 2 poles (11.5264, -48.6035) (11.5264, -48.6774) (11.4571, -48.7606) (11.3462, -48.7883) (11.2122, -48.7883) (11.1336, -48.7976) knots 0 0 0 1 2 3 4 4 4
  line L111 (11.1336, -48.7976) -> (7.1132, -49.0748)
  line L112 (7.1132, -49.0748) -> (6.1658, -49.0748)
  spline S116 degree 2 poles (6.1658, -49.0748) (6.1104, -49.0748) (6.0688, -49.0009) (6.0457, -48.9131) (6.0457, -48.8576) knots 0 0 0 1 2 3 3 3
  line L113 (6.0457, -48.8576) -> (6.0457, -48.7883)
  spline S117 degree 2 poles (6.0457, -48.7883) (6.0457, -48.6173) (6.2629, -48.4001) (6.4431, -48.4048) knots 0 0 0 1 2 2 2
  line L114 (11.8083, -45.0636) -> (11.6789, -45.0636)
  spline S118 degree 2 poles (11.6789, -45.0636) (11.6789, -45.0035) (11.7251, -44.8834) (11.8083, -44.8834) knots 0 0 0 1 2 2 2
  line L115 (11.8083, -44.8834) -> (11.8083, -45.0636)
  spline S119 degree 2 poles (6.7897, -45.2762) (6.7527, -45.2762) (6.6695, -45.2207) (6.6695, -45.1422) (6.7527, -45.0867) (6.7897, -45.0867) knots 0 0 0 1 2 3 4 4 4
  line L116 (6.7897, -45.0867) -> (6.7897, -45.2762)
  point P0 (0, 0)
  constraints: 2 other
extrude "Extrusion3" add sketch "Sketch4" along normal blind 0.5